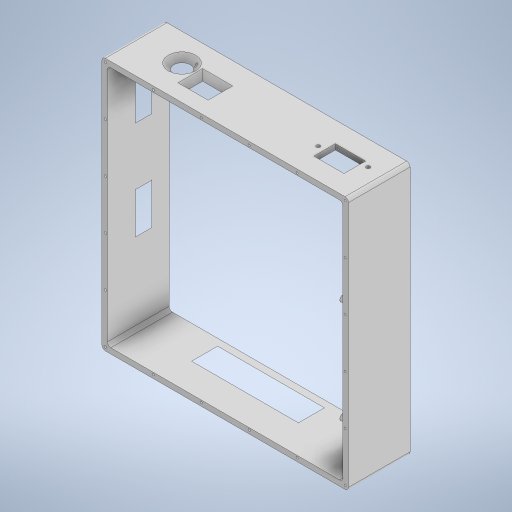
# Autodesk Inventor part: middle
Saved by Autodesk Inventor 2024 (Build 280153000, 153)
## iProperties
Created: 2023-05-28
Part Number: middle
Material: Generic
Document SubType Name: Modeling
Designer: elect
Density: 1 g/cm^3
Appearance: Default
Author: elect
Autodesk Inventor part; units mm, degrees
ref_plane "YZ Plane" through (0, 0, 0) normal (1, 0, 0) x (0, 1, 0)
ref_plane "XZ Plane" through (0, 0, 0) normal (0, 1, 0) x (-1, 0, 0)
ref_plane "XY Plane" through (0, 0, 0) normal (0, 0, 1) x (1, 0, 0)
sketch "Sketch1" plane through (0, 0, 0) normal (0, 0, 1) x (1, 0, 0)
  line L0 (-116.0602, 124.2038) -> (96.0298, 124.2038)
  line L1 (99.2048, 121.0288) -> (99.2048, -97.4112)
  line L2 (96.0298, -100.5862) -> (-116.0602, -100.5862)
  line L3 (-119.2352, -97.4112) -> (-119.2352, 121.0288)
  line L4 (-121.1402, 129.2838) -> (101.1098, 129.2838)
  line L5 (104.2848, 126.1088) -> (104.2848, -102.4912)
  line L6 (101.1098, -105.6662) -> (-121.1402, -105.6662)
  line L7 (-124.3152, -102.4912) -> (-124.3152, 126.1088)
  arc A0 (-121.1402, 129.2838) -> (-124.3152, 126.1088) centre (-121.1402, 126.1088) ccw
  arc A1 (-116.0602, 124.2038) -> (-119.2352, 121.0288) centre (-116.0602, 121.0288) ccw
  arc A2 (-124.3152, -102.4912) -> (-121.1402, -105.6662) centre (-121.1402, -102.4912) ccw
  arc A3 (-119.2352, -97.4112) -> (-116.0602, -100.5862) centre (-116.0602, -97.4112) ccw
  arc A4 (101.1098, -105.6662) -> (104.2848, -102.4912) centre (101.1098, -102.4912) ccw
  arc A5 (96.0298, -100.5862) -> (99.2048, -97.4112) centre (96.0298, -97.4112) ccw
  arc A6 (99.2048, 121.0288) -> (96.0298, 124.2038) centre (96.0298, 121.0288) ccw
  arc A7 (104.2848, 126.1088) -> (101.1098, 129.2838) centre (101.1098, 126.1088) ccw
  point P0 (0, 0)
  point P1 (104.2848, -105.6662)
  point P2 (104.2848, 129.2838)
  point P3 (-124.3152, -105.6662)
  dimension "d0" = 234.95
  dimension "d1" = 228.6
  dimension "d2" = 5.08
  dimension "d3" = 5.08
  dimension "d4" = 5.08
  dimension "d5" = 5.08
  dimension "d6" = 3.175
  constraints: 16 end point, 16 point on circle, 16 tangent, 8 centre point, 7 equal radius, 6 point on line, 4 parallel, 2 horizontal, 2 perpendicular
  measures "d0" distance of point (104.285, 129.284) point (104.285, -105.666)
  measures "d1" distance of point (104.285, -105.666) point (-124.315, -105.666)
  measures "d2" distance between parallel lines of L6 L2
  measures "d3" distance between parallel lines of L3 L7
  measures "d4" distance between parallel lines of L0 L4
  measures "d5" distance between parallel lines of L5 L1
  measures "d6" radius of A0
extrude "Extrusion1" add sketch "Sketch1" along normal blind 57.15
sketch "Sketch2" plane through (0, 0, 57.15) normal (0, 0, 1) x (1, 0, 0)
  arc A0 (-121.1402, 129.2838) -> (-124.3152, 126.1088) centre (-121.1402, 126.1088) ccw projected
  line L0 (-119.2352, -97.4112) -> (-119.2352, 121.0288) projected
  line L1 (-116.0602, 124.2038) -> (96.0298, 124.2038) projected
  point P0 (0, 0)
  point P1 (-121.1402, 80.3888)
  point P2 (-121.1402, 34.6688)
  point P3 (-121.1402, -11.0512)
  point P4 (-121.1402, -56.7712)
  point P5 (-121.1402, -102.4912)
  point P6 (-76.6902, -102.4912)
  point P7 (-32.2402, -102.4912)
  point P8 (12.2098, -102.4912)
  point P9 (56.6598, -102.4912)
  point P10 (101.1098, -102.4912)
  point P11 (-76.6902, 126.1088)
  point P12 (-32.2402, 126.1088)
  point P13 (12.2098, 126.1088)
  point P14 (56.6598, 126.1088)
  point P15 (101.1098, 126.1088)
  point P16 (101.1098, 80.3888)
  point P17 (101.1098, 34.6688)
  point P18 (101.1098, -11.0512)
  point P19 (101.1098, -56.7712)
  dimension "d11" = 45.72
  dimension "d18" = 44.45
  dimension "d25" = 44.45
  dimension "d32" = 45.72
  constraints: 2 horizontal, 2 vertical, 1 coincident, 19 other
  measures "d11" distance of point (-121.14, 126.109) point (-121.14, 80.389)
  measures "d18" distance of point (-121.14, -102.491) point (-76.69, -102.491)
  measures "d25" distance of point (-121.14, 126.109) point (-76.69, 126.109)
  measures "d32" distance of point (101.11, 126.109) point (101.11, 80.389)
hole "Hole1" at (-121.1402, 126.1088, 57.15) at (-121.1402, 80.3888, 57.15) at (-121.1402, 34.6688, 57.15) at (-121.1402, -11.0512, 57.15) at (-121.1402, -56.7712, 57.15) at (-121.1402, -102.4912, 57.15) at (-76.6902, -102.4912, 57.15) at (-32.2402, -102.4912, 57.15) at (12.2098, -102.4912, 57.15) at (56.6598, -102.4912, 57.15) at (101.1098, -102.4912, 57.15) at (-76.6902, 126.1088, 57.15) at (-32.2402, 126.1088, 57.15) at (12.2098, 126.1088, 57.15) at (56.6598, 126.1088, 57.15) at (101.1098, 126.1088, 57.15) at (101.1098, 80.3888, 57.15) at (101.1098, 34.6688, 57.15) at (101.1098, -11.0512, 57.15) at (101.1098, -56.7712, 57.15) direction (0, 0, -1) diameter 2.032 end through all
sketch "Sketch3" plane through (99.2048, -97.4112, 0) normal (-1, 0, 0) x (0, 0, 1)
  circle A0 centre (6.35, 42.545) radius 3
  circle A1 centre (50.8, 42.545) radius 3
  circle A2 centre (50.8, 137.795) radius 3
  circle A3 centre (6.35, 137.795) radius 3
  line L0 (57.15, -5.08) -> (57.15, 223.52) projected
  line L1 (0, -5.08) -> (0, 223.52) projected
  line L2 (0, -8.255) -> (57.15, -8.255) projected
  point P0 (0, 97.4112)
  dimension "d44" = 95.25
  dimension "d45" = 6
  dimension "d46" = 44.45
  dimension "d47" = 6.35
  dimension "d48" = 6.35
  dimension "d49" = 50.8
  constraints: 4 centre point, 3 equal radius, 2 horizontal alignment, 2 vertical alignment
  measures "d44" distance of A1.centre A2.centre
  measures "d45" diameter of A2
  measures "d46" distance of A2.centre A3.centre
  measures "d47" distance from line of L0 A2.centre
  measures "d48" distance from line of L1 A3.centre
  measures "d49" distance from line of L2 A1.centre
extrude "Extrusion2" add sketch "Sketch3" along normal blind 6.35
sketch "Sketch4" plane through (92.8548, 40.3838, 6.35) normal (-1, 0, 0) x (0, 0, 1)
  circle A0 centre (0, 0) radius 3 projected
  circle A1 centre (44.45, 0) radius 3 projected
  circle A2 centre (0, -95.25) radius 3 projected
  circle A3 centre (44.45, -95.25) radius 3 projected
  point P0 (-6.35, -40.3838)
  point P1 (44.45, 0)
  point P2 (0, -98.25)
  point P3 (0, -92.25)
  constraints: 4 coincident
hole "Hole2" at (92.8548, 40.3838, 6.35) at (92.8548, 40.3838, 50.8) at (92.8548, -54.8662, 6.35) at (92.8548, -54.8662, 50.8) direction (1, 0, 0) diameter 2.75 depth 6.35 tip angle 118
sketch "Sketch5" plane through (-121.1402, -105.6662, 0) normal (0, -1, 0) x (1, 0, 0)
  line L0 (53.34, 30.48) -> (152.4, 30.48)
  line L1 (152.4, 30.48) -> (152.4, 6.35)
  line L2 (152.4, 6.35) -> (53.34, 6.35)
  line L3 (53.34, 6.35) -> (53.34, 30.48)
  line L4 (0, 0) -> (222.25, 0) projected
  line L5 (0, 57.15) -> (222.25, 57.15) projected
  line L6 (222.25, 0) -> (222.25, 57.15) projected
  line L7 (0, 0) -> (0, 57.15) projected
  point P0 (121.1402, 0)
  point P1 (53.34, 18.415)
  dimension "d59" = 6.35
  dimension "d60" = 26.67
  dimension "d61" = 69.85
  dimension "d62" = 53.34
  constraints: 8 end point, 2 parallel, 1 horizontal, 1 midpoint, 1 perpendicular
  measures "d59" distance between parallel lines of L4 L2
  measures "d60" distance between parallel lines of L5 L0
  measures "d61" distance between parallel lines of L6 L1
  measures "d62" distance from line of L7 point (53.34, 18.415)
extrude "Extrusion3" cut sketch "Sketch5" against normal blind 6.35 contours L0 L1 L2 L3
sketch "Sketch6" plane through (-67.8002, -105.6662, 6.35) normal (0, 0, 1) x (1, 0, 0)
  circle A0 centre (35.56, 3.175) radius 1.016 projected
  circle A1 centre (80.01, 3.175) radius 1.016 projected
  point P0 (67.8002, 105.6662)
extrude "Extrusion4" add sketch "Sketch6" against normal blind 3.175
sketch "Sketch7" plane through (31.2598, -105.6662, 30.48) normal (0, 0, -1) x (-1, 0, 0)
  circle A0 centre (63.5, 3.175) radius 1.016 projected
  circle A1 centre (19.05, 3.175) radius 1.016 projected
  point P0 (31.2598, 105.6662)
extrude "Extrusion5" add sketch "Sketch7" against normal blind 3.175
chamfer "Chamfer1" distance 5.08 angle 45 4 edges at (-18.2702, -105.6662, 6.35) (-67.8002, -105.6662, 18.415) (-18.2702, -105.6662, 30.48) (31.2598, -105.6662, 18.415)
sketch "Sketch8" plane through (-124.3152, -102.4912, 0) normal (-1, 0, 0) x (0, 0, 1)
  line L0 (31.115, 205.74) -> (15.875, 205.74)
  line L1 (15.875, 205.74) -> (15.875, 167.64)
  line L2 (15.875, 167.64) -> (31.115, 167.64)
  line L3 (31.115, 167.64) -> (31.115, 205.74)
  line L4 (31.115, 114.3) -> (15.875, 114.3)
  line L5 (15.875, 114.3) -> (15.875, 76.2)
  line L6 (15.875, 76.2) -> (31.115, 76.2)
  line L7 (31.115, 76.2) -> (31.115, 114.3)
  line L8 (0, 228.6) -> (0, 0) projected
  line L9 (0, 228.6) -> (57.15, 228.6) projected
  point P0 (0, 102.4912)
  point P1 (23.495, 205.74)
  point P2 (23.495, 114.3)
  dimension "d73" = 15.875
  dimension "d74" = 15.875
  dimension "d75" = 22.86
  dimension "d76" = 53.34
  dimension "d77" = 38.1
  dimension "d78" = 38.1
  dimension "d81" = 15.24
  dimension "d82" = 15.24
  constraints: 16 end point, 5 equal length, 2 horizontal, 2 midpoint, 2 perpendicular
  measures "d73" distance between parallel lines of L8 L1
  measures "d74" distance between parallel lines of L8 L5
  measures "d75" distance from line of L9 point (23.495, 205.74)
  measures "d76" distance from line of point (23.495, 114.3) L2
  measures "d77" distance of L2.end L0.start
  measures "d78" distance of L6.end L4.start
  measures "d81" distance of L0.start L0.end
  measures "d82" distance of L4.start L4.end
extrude "Extrusion6" cut sketch "Sketch8" against normal up to surface (5.08 mm away)
sketch "Sketch9" plane through (-124.3152, 65.1488, 15.875) normal (0, 0, 1) x (1, 0, 0)
  circle A0 centre (3.175, 15.24) radius 1.016 projected
  circle A1 centre (3.175, -76.2) radius 1.016 projected
  circle A2 centre (3.175, -76.2) radius 1.016 projected
  line L0 (0, 38.1) -> (0, 0) projected
  circle A3 centre (3.175, 15.24) radius 1.016 projected
  point P0 (124.3152, -65.1488)
extrude "Extrusion7" add sketch "Sketch9" against normal blind 3.175
sketch "Sketch11" plane through (-124.3152, 65.1488, 31.115) normal (0, 0, -1) x (-1, 0, 0)
  circle A0 centre (-3.175, 15.24) radius 1.016 projected
  circle A1 centre (-3.175, -76.2) radius 1.016 projected
  point P0 (-124.3152, -65.1488)
extrude "Extrusion8" add sketch "Sketch11" against normal blind 3.175
chamfer "Chamfer2" distance 5.08 angle 45 8 edges at (-124.3152, 84.1988, 31.115) (-124.3152, 103.2488, 23.495) (-124.3152, 84.1988, 15.875) (-124.3152, 65.1488, 23.495) (-124.3152, 11.8088, 23.495) (-124.3152, -7.2412, 31.115) (-124.3152, -7.2412, 15.875) (-124.3152, -26.2912, 23.495)
sketch "Sketch12" plane through (-121.1402, 129.2838, 0) normal (0, 1, 0) x (1, 0, 0)
  circle A0 centre (39.37, -25.4) radius 7.62
  line L0 (0, 0) -> (0, -57.15) projected
  line L1 (222.25, -57.15) -> (0, -57.15) projected
  line L2 (76.2, -38.1) -> (58.42, -38.1)
  line L3 (58.42, -38.1) -> (58.42, -25.4)
  line L4 (58.42, -25.4) -> (76.2, -25.4)
  line L5 (76.2, -25.4) -> (76.2, -38.1)
  point P0 (121.1402, 0)
  point P1 (58.42, -31.75)
  dimension "d90" = 15.24
  dimension "d94" = 39.37
  dimension "d95" = 31.75
  dimension "d96" = 12.7
  dimension "d97" = 17.78
  dimension "d98" = 19.05
  dimension "d128" = 19.05
  constraints: 8 end point, 2 parallel, 1 centre point, 1 horizontal, 1 midpoint, 1 perpendicular
  measures "d90" diameter of A0
  measures "d94" distance from line of L0 A0.centre
  measures "d95" distance from line of L1 A0.centre
  measures "d96" distance of L4.end L2.start
  measures "d97" distance of L2.start L2.end
  measures "d98" distance from line of A0.centre L3
  measures "d128" distance between parallel lines of L1 L2
extrude "Extrusion9" cut sketch "Sketch12" against normal up to surface (5.08 mm away)
chamfer "Chamfer4" distance 5.08 angle 45 5 edges at (-53.8302, 129.2838, 38.1) (-44.9402, 129.2838, 31.75) (-53.8302, 129.2838, 25.4) (-62.7202, 129.2838, 31.75) (-89.3902, 129.2838, 25.4)
sketch "Sketch14" plane through (-121.1402, 129.2838, 0) normal (0, 1, 0) x (1, 0, 0)
  line L0 (175.2092, -39.0398) -> (203.2, -39.0398)
  line L1 (203.2, -39.0398) -> (203.2, -19.05)
  line L2 (203.2, -19.05) -> (175.2092, -19.05)
  line L3 (175.2092, -19.05) -> (175.2092, -39.0398)
  line L4 (222.25, 0) -> (0, 0) projected
  line L5 (222.25, -57.15) -> (0, -57.15) projected
  line L6 (222.25, 0) -> (222.25, -57.15) projected
  point P0 (121.1402, 0)
  point P1 (189.2046, -39.0398)
  point P2 (169.2148, -29.0449)
  point P3 (209.1944, -22.6949)
  point P4 (175.2092, -29.0449)
  dimension "d112" = 27.9908
  dimension "d113" = 19.9898
  dimension "d114" = 19.05
  dimension "d115" = 18.1102
  dimension "d116" = 19.05
  dimension "d117" = 5.9944
  dimension "d118" = 5.9944
  constraints: 8 end point, 2 midpoint, 2 parallel, 1 horizontal, 1 perpendicular
  measures "d112" distance of L0.start L0.end
  measures "d113" distance of L2.end L0.start
  measures "d114" distance between parallel lines of L4 L2
  measures "d115" distance from line of L5 point (189.205, -39.04)
  measures "d116" distance between parallel lines of L6 L1
  measures "d117" distance from line of L1 point (209.194, -22.695)
  measures "d118" distance of point (175.209, -29.045) point (169.215, -29.045)
extrude "Extrusion11" cut sketch "Sketch14" against normal blind 25.4
hole "Hole3" at (48.0746, 129.2838, 29.0449) at (88.0542, 129.2838, 22.6949) direction (0, -1, 0) diameter 3.5 depth 6.35 tip angle 118
body "Solid1"
